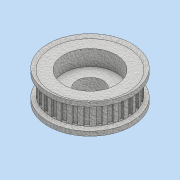
# Autodesk Inventor part: Koło zębate 21 T5 28 2F
Saved by Autodesk Inventor 2018 (Build 220112000, 112)
## iProperties
Created: 2019-01-25
Part Number: Koło zębate 21 T5 28 2F
Material: Ogólny
Document SubType Name: Modeling
Designer: Dawid
Density: 1 g/cm^3
Appearance: Aluminium odlewane
Author: Dawid
Autodesk Inventor part; units mm, degrees
ref_plane "YZ Plane" through (0, 0, 0) normal (1, 0, 0) x (0, 1, 0)
ref_plane "XZ Plane" through (0, 0, 0) normal (0, 1, 0) x (-1, 0, 0)
ref_plane "XY Plane" through (0, 0, 0) normal (0, 0, 1) x (1, 0, 0)
sketch "Szkic1" plane through (0, 0, 0) normal (0, 0, 1) x (1, 0, 0)
  arc A0 (2.4494, 21.7374) -> (0, 21.875) centre (0, 0) ccw
  line L0 (0, 21.875) -> (0, 0)
  line L1 (0, 0) -> (2.4494, 21.7374)
  line L2 (0, 0) -> (25.5388, 0) construction
  line L3 (0, 21.875) -> (0, 20.675)
  arc A1 (0, 20.675) -> (2.315, 20.545) centre (0, 0) ccw
  constraints: 8 end point, 4 point on circle, 2 centre point, 2 coincident, 2 point on line
extrude "Wyciągnięcie proste1" add sketch "Szkic1" along normal blind 15
pattern_circular "Szyk kołowy1" count 28 over 360 about axis through (0, 0, 0) along (0, 0, 1) of "Wyciągnięcie proste1"
sketch "Szkic2" plane through (0, 0, 0) normal (0, 0, -1) x (-1, 0, 0)
  circle A0 centre (0, 0) radius 16
  dimension "d12" = 32
  constraints: 1 centre point, 1 coincident
  measures "d12" diameter of A0
extrude "Wyciągnięcie proste2" add sketch "Szkic2" along normal blind 6
sketch "Szkic3" plane through (0, 0, 0) normal (1, 0, 0) x (0, 1, 0)
  line L0 (0, 15) -> (-2.3147, 15) projected
  line L1 (0, 15) -> (21.875, 15)
  line L2 (24, 15) -> (24, 0)
  line L3 (2.4494, 0) -> (0, 0) projected
  line L4 (21.875, 0) -> (0, 0)
  line L5 (0, 0) -> (0, 15)
  line L6 (24, 0) -> (24, -1)
  line L7 (24, -1) -> (21.875, 0)
  line L8 (0, 0) -> (0, 2.5)
  line L9 (0, 2.5) -> (21.875, 2.5)
  line L10 (24, 2.5) -> (24, 1.5)
  line L11 (21.875, 2.5) -> (24, 1.5)
  line L12 (24, 15) -> (24, 16)
  line L13 (24, 16) -> (21.875, 15)
  line L14 (24, 12.5) -> (24, 13.5)
  line L15 (24, 13.5) -> (21.875, 12.5)
  line L16 (21.875, 12.5) -> (0, 12.5)
  dimension "d18" = 2.5
  constraints: 30 end point, 6 point on line, 5 perpendicular, 2 vertical, 1 horizontal
  measures "d18" distance of L3.end L8.end
revolve "Obrót1" add sketch "Szkic3" angle 360 about axis through (0, 0, 0) along (0, 0, 1) contours L1 L13 L12 L2 L15 L16 L5 | L9 L11 L2 L6 L7 L4 L3 L5
sketch "Szkic4" plane through (0, 0, -6) normal (0, 0, -1) x (-1, 0, 0)
  circle A0 centre (0, 0) radius 7.5
  dimension "d26" = 15
  constraints: 1 centre point, 1 coincident
  measures "d26" diameter of A0
extrude "Wyciągnięcie proste3" cut sketch "Szkic4" against normal up to next
sketch "Szkic6" plane through (0, 0, 15) normal (0, 0, 1) x (1, 0, 0)
  circle A0 centre (0, 0) radius 15
  circle A1 centre (0, 0) radius 7.5 projected
  dimension "d32" = 30
  constraints: 1 centre point, 1 coincident
  measures "d32" diameter of A0
extrude "Wyciągnięcie proste5" cut sketch "Szkic6" against normal blind 9
